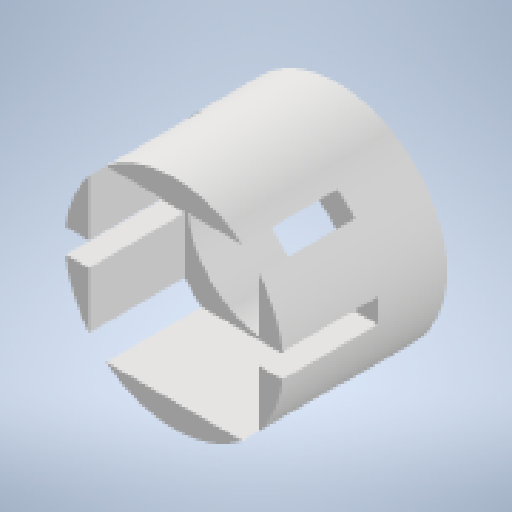
# Autodesk Inventor part: CouplerAdapter
Saved by Autodesk Inventor 2023.1 (Build 271208000, 208)
## iProperties
Created: 2023-06-07
Part Number: CouplerAdapter
Material: Generic
Document SubType Name: Modeling
Designer: hello
Density: 1 g/cm^3
Appearance: Default
Author: hello
Autodesk Inventor part; units mm, degrees
ref_plane "YZ Plane" through (0, 0, 0) normal (1, 0, 0) x (0, 1, 0)
ref_plane "XZ Plane" through (0, 0, 0) normal (0, 1, 0) x (-1, 0, 0)
ref_plane "XY Plane" through (0, 0, 0) normal (0, 0, 1) x (1, 0, 0)
sketch "Sketch1" plane through (0, 0, 0) normal (0, 0, 1) x (1, 0, 0)
  circle A0 centre (0, 0) radius 7.975
  circle A1 centre (0, 0) radius 6.05
  dimension "d0" = 15.95
  dimension "d1" = 12.1
  constraints: 2 centre point, 2 coincident
  measures "d0" diameter of A0
  measures "d1" diameter of A1
extrude "Extrusion1" add sketch "Sketch1" along normal blind 10
sketch "Sketch2" plane through (0, 0, 10) normal (0, 0, 1) x (1, 0, 0)
  circle A0 centre (0, 0) radius 7.975 projected
  line L0 (-6.225, 6.225) -> (6.225, 6.225)
  line L1 (6.225, 6.225) -> (6.225, -6.225)
  line L2 (6.225, -6.225) -> (-6.225, -6.225)
  line L3 (-6.225, -6.225) -> (-6.225, 6.225)
  line L4 (-6.225, 6.225) -> (6.225, -6.225) construction
  line L5 (6.225, 6.225) -> (-6.225, -6.225) construction
  line L6 (-8.5, 0.875) -> (8.5, 0.875)
  line L7 (8.5, 0.875) -> (8.5, -0.875)
  line L8 (8.5, -0.875) -> (-8.5, -0.875)
  line L9 (-8.5, -0.875) -> (-8.5, 0.875)
  line L10 (-8.5, 0.875) -> (8.5, -0.875) construction
  line L11 (8.5, 0.875) -> (-8.5, -0.875) construction
  circle A1 centre (0, 0) radius 12
  point P0 (4.985, -6.225)
  point P1 (-4.985, -6.225)
  point P2 (7.9269, -0.875)
  point P3 (6.225, -0.875)
  point P4 (6.225, -4.985)
  point P5 (-6.225, -0.875)
  point P6 (-7.9269, -0.875)
  point P7 (-6.225, -4.985)
  point P8 (6.225, 0.875)
  point P9 (7.9269, 0.875)
  point P10 (6.225, 4.985)
  point P11 (-7.9269, 0.875)
  point P12 (-6.225, 0.875)
  point P13 (-6.225, 4.985)
  point P14 (-4.985, 6.225)
  point P15 (4.985, 6.225)
  dimension "d4" = 12.45
  dimension "d5" = 12.45
  dimension "d6" = 17
  dimension "d7" = 1.75
  dimension "d10" = 24
  constraints: 24 end point, 4 midpoint, 4 parallel, 2 horizontal, 2 perpendicular, 1 centre point, 1 coincident
  measures "d4" distance of L1.end L2.end
  measures "d5" distance of L0.end L1.end
  measures "d6" distance of L7.end L8.end
  measures "d7" distance of L6.end L7.end
  measures "d10" diameter of A1
extrude "Extrusion2" add sketch "Sketch2" along normal blind 7 contours L6 L1 A0 | A0 L1 L8 | L0 A0 | L6 A0 L3 | A0 L2 | L3 A0 L8 | A1
sketch "Sketch3" plane through (0, 0, 10) normal (0, 0, -1) x (-1, 0, 0)
  circle A0 centre (0, 0) radius 7.975 projected
  circle A1 centre (0, 0) radius 12 projected
extrude "Extrusion3" add sketch "Sketch3" along normal blind 0.2
chamfer "Chamfer1" distance 2 angle 45 1 edges at (-7.975, 0, 9.8)
chamfer "Chamfer2" distance 2 angle 45 1 edges at (12, 0, 9.8)
body "Solid1"
